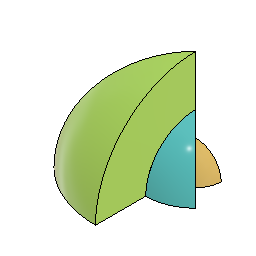
03-Refinements (Autodesk Fusion 360 design; units mm, degrees)
Autodesk Fusion 360 part; units mm, degrees
sketch "Sketch2" plane through (0, 0, 0) normal (0, 0, 1) x (1, 0, 0)
  circle A0 centre (0, 0) radius 200
  line L0 (0, 200) -> (0, -200)
  line L1 (-200, 0) -> (200, 0)
  line L2 (-141.4214, 141.4214) -> (141.4214, -141.4214)
  line L3 (-141.4214, -141.4214) -> (141.4214, 141.4214)
  line L4 (0, -200) -> (0, 200)
  line L5 (-200, 0) -> (200, 0)
  circle A1 centre (0, 0) radius 50
  circle A2 centre (0, 0) radius 100
  dimension "d7" = 400
  dimension "d8" = 45
  dimension "d9" = 45
  dimension "d10" = 100
  dimension "d11" = 200
  constraint coincident A0.centre A1.centre
  constraint coincident A0 L0.start
  constraint coincident A0 L0.end
  constraint vertical L0
  constraint coincident A0 L1.start
  constraint coincident A0 L1.end
  constraint perpendicular L0 L1
  constraint coincident A0 L2.start
  constraint coincident A0 L2.end
  constraint coincident A0 L3.start
  constraint coincident A0 L3.end
  constraint midpoint A0.centre L3
  constraint midpoint A0.centre L2
  constraint parallel L0 L4
  constraint midpoint A0.centre L1
  constraint concentric A0 A1
  constraint concentric A1 A2
  measures "d7" diameter of A0
  measures "d8" angle of L0 L2
  measures "d9" angle of L0 L3
  measures "d10" diameter of A1
  measures "d11" diameter of A2
extrude "Extrude1" add sketch "Sketch2" along normal blind 50 contours L1 L2 L5 A1 picked at (27.6563, -18.4794) makes body 1 in component "Small"
extrude "Extrude1'" add sketch "Sketch2" along normal blind 100 separate body contours L0 L2 L4 A1 A2 | L0 L2 L4 A1 picked at (55.6474, -61.8005) picked at (10.6917, -31.4968) makes body 2 in component "Medium"
extrude "Extrude1''" add sketch "Sketch2" along normal blind 200 separate body contours A0 L0 L3 L4 A2 | L0 L3 L4 A1 A2 | L0 L3 L4 A1 picked at (-8.7017, -166.0963) picked at (-37.7561, -74.0973) picked at (-10.6917, -31.4968) makes body 3 in component "Large"
fillet "Fillet1" radius 50 1 edges at (46.194, -19.1342, 50) on bodies 1 in component "Small"
fillet "Fillet2" radius 100 1 edges at (38.2683, -92.388, 100) on bodies 2 in component "Medium"
fillet "Fillet1'" radius 200 1 edges at (-76.5367, -184.7759, 200) on bodies 3 in component "Large"
revolve "Revolve1" cut 1 faces at (23.461, -23.461, 2.2699) angle 180 about axis through (0, 0, 1.75) along (0, 0, -1) on bodies 1 bodies 2 in component "Medium"
revolve "Revolve1'" cut 1 faces at (23.461, -23.461, 2.2699) angle 180 about axis through (0, 0, 1.75) along (0, 0, -1) on bodies 1 bodies 3 in component "Large"
revolve "Revolve2" cut 1 faces at (0, -37.0989, 74.4235) angle 180 about axis through (0, 0, 1.75) along (0, 0, -1) on bodies 2 bodies 3 in component "Large"
component "Small" placed x (1, 0, 0) y (0, 1, 0) z (0, 0, 1) at (0, 0, 0)
component "Medium" placed x (1, 0, 0) y (0, 1, 0) z (0, 0, 1) at (0, 0, 0)
component "Large" placed x (1, 0, 0) y (0, 1, 0) z (0, 0, 1) at (0, 0, 0)
